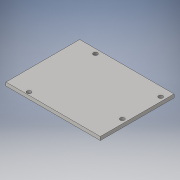
# Autodesk Inventor part: arduino uno model
Saved by Autodesk Inventor 2016 (Build 200138000, 138)
## iProperties
Created: 2017-09-27
Part Number: arduino uno model
Material: Generic
Document SubType Name: Modeling
Designer: Student
Density: 1 g/cm^3
Appearance: Default
Author: Student
Autodesk Inventor part; units mm, degrees
ref_plane "YZ Plane" through (0, 0, 0) normal (1, 0, 0) x (0, 1, 0)
ref_plane "XZ Plane" through (0, 0, 0) normal (0, 1, 0) x (-1, 0, 0)
ref_plane "XY Plane" through (0, 0, 0) normal (0, 0, 1) x (1, 0, 0)
sketch "Sketch1" plane through (0, 0, 0) normal (0, 1, 0) x (-1, 0, 0)
  line L0 (34.4209, 32.9812) -> (-34.1591, 32.9812)
  line L1 (-34.1591, 32.9812) -> (-34.1591, -20.6128)
  line L2 (-34.1591, -20.6128) -> (34.4209, -20.6128)
  line L3 (34.4209, -20.6128) -> (34.4209, 32.9812)
  circle A0 centre (19.6889, 30.9492) radius 1.524
  circle A1 centre (19.6889, -17.3108) radius 1.524
  circle A2 centre (-31.1111, -14.0088) radius 1.524
  circle A3 centre (-31.1111, 13.9312) radius 1.524
  point P0 (0, 0)
  dimension "d0" = 68.58
  dimension "d1" = 53.594
  dimension "d2" = 14.732
  dimension "d3" = 2.032
  dimension "d4" = 3.048
  dimension "d5" = 48.26
  dimension "d6" = 6.604
  dimension "d7" = 3.048
  dimension "d8" = 27.94
  constraints: 8 end point, 4 centre point, 2 equal radius, 2 parallel, 1 horizontal, 1 perpendicular
  measures "d0" distance of L0.start L0.end
  measures "d1" distance of L2.end L0.start
  measures "d2" distance from line of L3 A0.centre
  measures "d3" distance from line of L0 A0.centre
  measures "d4" diameter of A0
  measures "d5" distance of A1.centre A0.centre
  measures "d6" distance from line of L2 A2.centre
  measures "d7" distance from line of L1 A2.centre
  measures "d8" distance of A2.centre A3.centre
extrude "Extrusion1" add sketch "Sketch1" along normal blind 2.54
body "Solid1"
